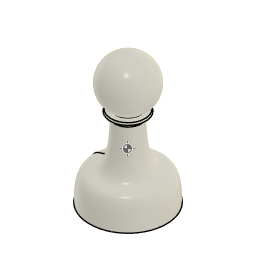
Pawn v2 (Autodesk Fusion 360 design; units mm, degrees)
Autodesk Fusion 360 part; units mm, degrees
sketch "Sketch1" plane through (0, 0, 0) normal (0, 1, 0) x (1, 0, 0)
  line L0 (0, 0) -> (-15, 0)
  spline S0 degree 5 poles (-15, 0) (-15, -2.4594) (-14.7958, -6.5576) (-13.8775, -10.2456) (-11.6701, -11.3146) (-8.3299, -11.1548) (-6.1225, -14.3711) (-5.2042, -21.1026) (-5, -27.9377) (-5, -31.9428) knots 0 0 0 0 0 0 0.2 0.4 0.6 0.8 1 1 1 1 1 1
  line L1 (-15, 5) -> (-15, -5)
  line L2 (0, 0) -> (0, -50)
  line L3 (-5, -23.8005) -> (-5, -40.085)
  line L4 (-5, -31.9428) -> (-6.6248, -31.4797)
  line L5 (-6.9086, -30.7495) -> (-5.0265, -28.8674)
  arc A0 (0, -30.5583) -> (0, -50) centre (0, -40.2791) ccw
  line L6 (-6.6248, -31.4797) -> (-6.9086, -30.7495)
  dimension "d2" = 15
  dimension "d4" = 50
  dimension "d5" = 45
  dimension "d10" = 5
  constraint coincident L0.start L2.start
  constraint horizontal L0
  constraint midpoint L0.end L1
  constraint vertical L1
  constraint perpendicular L0 L2
  constraint midpoint S0.end L3
  constraint vertical L3
  constraint coincident S0 L4.start
  constraint coincident S0 L5.end
  constraint coincident L2 A0.start
  constraint coincident L2 A0.centre
  constraint coincident S0.end A0
  constraint coincident L3 S0.end
  measures "d2" distance of L0.start L0.end
  measures "d4" distance of L0.start L2.end
  measures "d5" angle of L3 L5
  measures "d10" distance of L2 L3
revolve "Revolve1" add sketch "Sketch1" angle 360 about axis through (0, 0, 0) along (0, 0, 1)
equation "d2 = 1 / 2 * 3 cm"
